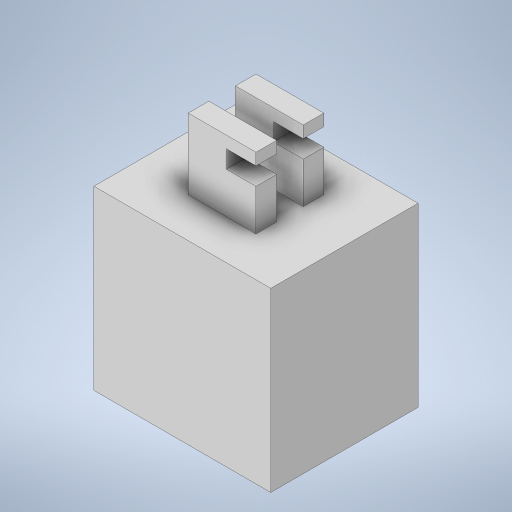
# Autodesk Inventor part: base
Saved by Autodesk Inventor 2024.3 (Build 283343000, 343)
## iProperties
Created: 2024-10-09
Part Number: base
Material: Generic
Document SubType Name: Modeling
Designer: pjcaa
Density: 1 g/cm^3
Appearance: Default
Author: pjcaa
Autodesk Inventor part; units mm, degrees
ref_plane "YZ Plane" through (0, 0, 0) normal (1, 0, 0) x (0, 1, 0)
ref_plane "XZ Plane" through (0, 0, 0) normal (0, 1, 0) x (-1, 0, 0)
ref_plane "XY Plane" through (0, 0, 0) normal (0, 0, 1) x (1, 0, 0)
sketch "Sketch12" plane through (0, 0, 0) normal (0, 0, 1) x (1, 0, 0)
  line L0 (-12.5, 15) -> (12.5, 15)
  line L1 (12.5, 15) -> (12.5, -15)
  line L2 (12.5, -15) -> (-12.5, -15)
  line L3 (-12.5, -15) -> (-12.5, 15)
  line L4 (-12.5, 15) -> (12.5, -15) construction
  line L5 (12.5, 15) -> (-12.5, -15) construction
  point P0 (0, 0)
  dimension "d48" = 25
  dimension "d49" = 30
  constraints: 12 end point, 2 midpoint, 2 parallel, 1 horizontal, 1 perpendicular
  measures "d48" distance of L1.end L2.end
  measures "d49" distance of L0.end L1.end
extrude "Extrusion12" add sketch "Sketch12" along normal blind 30
sketch "Sketch14" plane through (0, 0, 0) normal (0, 0, -1) x (-1, 0, 0)
  circle A0 centre (0, 0) radius 10.75
  dimension "d71" = 21.5
  constraints: 1 centre point, 1 coincident
  measures "d71" diameter of A0
extrude "Extrusion14" cut sketch "Sketch14" against normal blind 28
sketch "Sketch15" plane through (0, 0, 30) normal (0, 0, 1) x (1, 0, 0)
  line L0 (5.75, 5.75) -> (-5.75, 5.75) construction
  line L1 (-5.75, 5.75) -> (-5.75, -5.75) construction
  line L2 (-5.75, -5.75) -> (5.75, -5.75) construction
  line L3 (5.75, -5.75) -> (5.75, 5.75) construction
  line L4 (5.75, 5.75) -> (-5.75, -5.75) construction
  line L5 (-5.75, 5.75) -> (5.75, -5.75) construction
  line L6 (5.75, 5.75) -> (2.25, 5.75)
  line L7 (2.25, 5.75) -> (2.25, -5.75)
  line L8 (2.25, -5.75) -> (5.75, -5.75)
  line L9 (5.75, -5.75) -> (5.75, 5.75)
  line L10 (-5.75, 5.75) -> (-2.25, 5.75)
  line L11 (-2.25, 5.75) -> (-2.25, -5.75)
  line L12 (-2.25, -5.75) -> (-5.75, -5.75)
  line L13 (-5.75, -5.75) -> (-5.75, 5.75)
  point P0 (0, 0)
  dimension "d74" = 11.5
  dimension "d75" = 11.5
  dimension "d76" = 3.5
  dimension "d78" = 3.5
  constraints: 28 end point, 8 parallel, 3 horizontal, 3 perpendicular, 2 midpoint
  measures "d74" distance of L2.end L1.end
  measures "d75" distance of L1.end L0.end
  measures "d76" distance of L8.end L7.end
  measures "d78" distance of L11.end L12.end
extrude "Extrusion15" add sketch "Sketch15" along normal blind 12
sketch "Sketch16" plane through (-5.75, -5.75, 30) normal (0, -1, 0) x (1, 0, 0)
  line L0 (8, 0) -> (11.5, 0) construction
  line L1 (8, 0) -> (8, 12) construction
  line L2 (11.5, 12) -> (8, 12) construction
  line L3 (11.5, 0) -> (11.5, 12) construction
  line L4 (0, 0) -> (3.5, 0) construction
  line L5 (0, 0) -> (0, 12) construction
  line L6 (3.5, 12) -> (0, 12) construction
  line L7 (3.5, 0) -> (3.5, 12) construction
  line L8 (0, 10) -> (11.5, 10)
  line L9 (11.5, 10) -> (11.5, 7)
  line L10 (11.5, 7) -> (0, 7)
  line L11 (0, 7) -> (0, 10)
  point P0 (5.75, -30)
  dimension "d82" = 2
  dimension "d83" = 3
  constraints: 8 end point, 2 parallel, 2 point on line, 1 horizontal, 1 perpendicular
  measures "d82" distance between parallel lines of L8 L2
  measures "d83" distance between parallel lines of L8 L10
extrude "Extrusion16" cut sketch "Sketch16" against normal blind 5
body "Solid2"
